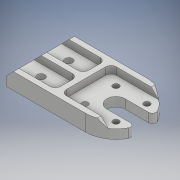
# Autodesk Inventor part: holder-LMF8LUU-z-axis-v2
Saved by Autodesk Inventor 2018 (Build 220112000, 112)
## iProperties
Created: 2017-12-27
Part Number: holder-LMF8LUU-z-axis-v2
Material: Generic
Document SubType Name: Modeling
Designer: Jurjen
Density: 1 g/cm^3
Appearance: Default
Author: Jurjen
Autodesk Inventor part; units mm, degrees
ref_plane "YZ Plane" through (0, 0, 0) normal (1, 0, 0) x (0, 1, 0)
ref_plane "XZ Plane" through (0, 0, 0) normal (0, 1, 0) x (-1, 0, 0)
ref_plane "XY Plane" through (0, 0, 0) normal (0, 0, 1) x (1, 0, 0)
sketch "Sketch1" plane through (0, 0, 0) normal (0, 0, 1) x (1, 0, 0)
  arc A0 (13.75, 5) -> (13.75, -5) centre (13.75, 0) ccw
  line L0 (29.75, 16.75) -> (-29.75, 16.75)
  line L1 (-29.75, 16.75) -> (-29.75, -16.75)
  line L2 (-29.75, -16.75) -> (29.75, -16.75)
  line L3 (29.75, -16.75) -> (29.75, 16.75)
  line L4 (13.75, 5) -> (29.75, 5)
  line L5 (13.75, -5) -> (29.75, -5)
  arc A1 (13.75, -5) -> (13.75, 5) centre (13.75, 0) ccw construction
  point P0 (0, 0)
  point P1 (0, -16.75)
  point P2 (29.75, 0)
  point P3 (-29.75, 0)
  dimension "d0" = 10
  dimension "d1" = 33.5
  dimension "d2" = 16
  dimension "d3" = 43.5
  constraints: 12 end point, 4 point on circle, 3 midpoint, 3 perpendicular, 2 centre point, 2 horizontal alignment, 2 parallel, 2 point on line, 2 tangent, 1 horizontal, 1 vertical alignment
  measures "d0" diameter of A0
  measures "d1" distance between parallel lines of L2 L0
  measures "d2" distance from line of L3 A0.centre
  measures "d3" distance from line of L1 A0.centre
extrude "Extrusion1" add sketch "Sketch1" along normal mid plane 5 contours A0 L5 L3 L2 L1 L0 L4
sketch "Sketch2" plane through (0, 0, 2.5) normal (0, 0, 1) x (1, 0, 0)
  arc A0 (13.75, 5) -> (13.75, -5) centre (13.75, 0) ccw projected
  circle A1 centre (5.2647, 8.4853) radius 1.65
  line L0 (13.75, 0) -> (5.2647, 8.4853) construction
  line L1 (13.75, 0) -> (0, 0) construction
  line L2 (13.75, 0) -> (13.75, -13.75) construction
  circle A2 centre (5.2647, -8.4853) radius 1.65
  line L3 (13.75, 0) -> (27.5, 0) construction
  circle A3 centre (22.2353, -8.4853) radius 1.65
  line L4 (13.75, 0) -> (13.75, 13.75) construction
  circle A4 centre (22.2353, 8.4853) radius 1.65
  dimension "d6" = 45
  dimension "d7" = 12
  dimension "d8" = 3.3
  dimension "d11" = 360
  constraints: 10 end point, 4 centre point, 2 coincident, 1 horizontal, 19 other
  measures "d6" angle of L1 L0
  measures "d7" distance of L0.start L0.end
  measures "d8" diameter of A1
extrude "Extrusion2" cut sketch "Sketch2" against normal through all
sketch "Sketch3" plane through (0, 0, 2.5) normal (0, 0, 1) x (1, 0, 0)
  circle A0 centre (-19.75, 7.625) radius 2.1
  line L0 (0, 0) -> (-29.75, 0) construction
  line L1 (-29.75, 16.75) -> (-29.75, -16.75) projected
  circle A1 centre (-19.75, -7.625) radius 2.1
  dimension "d15" = 4.2
  dimension "d16" = 10
  dimension "d37" = 9.125
  constraints: 2 centre point, 2 end point, 1 midpoint, 1 symmetric about line, 1 other
  measures "d15" diameter of A0
  measures "d16" distance from line of A0.centre L1
  measures "d37" vertical distance of A0.centre L1.start
extrude "Extrusion3" cut sketch "Sketch3" against normal through all
sketch "Sketch4" plane through (0, 0, 2.5) normal (0, 0, 1) x (1, 0, 0)
  line L0 (-29.75, 16.75) -> (29.75, 16.75) projected
  line L1 (-29.75, 16.75) -> (29.75, 16.75)
  line L2 (29.75, 16.75) -> (29.75, 13.75)
  line L3 (-29.75, 13.75) -> (-29.75, 16.75)
  line L4 (-2.75, 13.75) -> (-2.75, 0)
  line L5 (-5.75, 1.5) -> (-5.75, 13.75)
  line L6 (-29.75, 1.5) -> (-5.75, 1.5)
  line L7 (-29.75, 0) -> (-29.75, 1.5)
  line L8 (29.75, 13.75) -> (-2.75, 13.75)
  line L9 (-5.75, 13.75) -> (-29.75, 13.75)
  line L10 (0, 0) -> (-29.75, 0) construction
  line L11 (-29.75, -16.75) -> (-29.75, 16.75) projected
  line L12 (-29.75, -16.75) -> (29.75, -16.75)
  line L13 (-29.75, -16.75) -> (29.75, -16.75)
  line L14 (29.75, -16.75) -> (29.75, -13.75)
  line L15 (-29.75, -13.75) -> (-29.75, -16.75)
  line L16 (-2.75, -13.75) -> (-2.75, 0)
  line L17 (-5.75, -1.5) -> (-5.75, -13.75)
  line L18 (-29.75, -1.5) -> (-5.75, -1.5)
  line L19 (-29.75, 0) -> (-29.75, -1.5)
  line L20 (29.75, -13.75) -> (-2.75, -13.75)
  line L21 (-5.75, -13.75) -> (-29.75, -13.75)
  point P0 (29.75, 5)
  dimension "d20" = 3
  dimension "d21" = 3
  dimension "d23" = 24
  dimension "d24" = 1.5
  constraints: 40 end point, 8 symmetric about line, 5 parallel, 3 horizontal alignment, 3 perpendicular, 2 horizontal, 2 point on line, 2 vertical alignment
  measures "d20" distance between parallel lines of L0 L8
  measures "d21" distance between parallel lines of L4 L5
  measures "d23" distance of L5.end L3.start
  measures "d24" distance of L7.start L6.start
extrude "Extrusion4" add sketch "Sketch4" along normal blind 4 contours L0 L2 L8 L4 L16 L20 L14 L12 L11 L21 L17 L18 L7 L6 L5 L9 L3
sketch "Sketch5" plane through (0, 0, -2.5) normal (0, 0, -1) x (-1, 0, 0)
  arc A0 (-13.75, -5) -> (-13.75, 5) centre (-13.75, 0) ccw projected
  line L0 (29.75, 16.75) -> (-29.75, 16.75) projected
  circle A1 centre (19.75, 7.625) radius 2.1 projected
  circle A2 centre (19.75, -7.625) radius 2.1 projected
  circle A3 centre (-22.2353, -8.4853) radius 1.65 projected
  circle A4 centre (-5.2647, 8.4853) radius 1.65 projected
  circle A5 centre (-5.2647, -8.4853) radius 1.65 projected
  circle A6 centre (-22.2353, 8.4853) radius 1.65 projected
  line L1 (29.75, 16.75) -> (-29.75, 16.75) projected
  line L2 (-29.75, 16.75) -> (-29.75, 5) projected
  line L3 (-29.75, 5) -> (-13.75, 5) projected
  arc A7 (-13.75, -5) -> (-13.75, 5) centre (-13.75, 0) ccw projected
  line L4 (-13.75, -5) -> (-29.75, -5) projected
  line L5 (-29.75, -5) -> (-29.75, -16.75) projected
  line L6 (-29.75, -16.75) -> (29.75, -16.75) projected
  line L7 (29.75, -16.75) -> (29.75, 16.75) projected
  line L8 (-13.75, -16.75) -> (-29.75, -16.75)
  line L9 (-29.75, -13.75) -> (-29.75, -5) projected
  line L10 (-29.75, -5) -> (-29.75, -16.75)
  line L11 (-29.75, 5) -> (-29.75, 16.75)
  line L12 (-13.75, 16.75) -> (-29.75, 16.75)
  arc A8 (-13.75, 16.75) -> (-29.7363, 5) centre (-13.75, 0) ccw
  arc A9 (-29.7363, -5) -> (-13.75, -16.75) centre (-13.75, 0) ccw
  point P0 (0, 0)
  constraints: 8 end point, 4 point on circle, 4 point on line, 3 collinear, 2 centre point, 2 tangent, 1 coincident, 1 perpendicular
extrude "Extrusion5" cut sketch "Sketch5" against normal through all contours A9 L6 L5 L4 | L3 L2 L0 A8
fillet "Fillet1" radius 2 2 edges at (29.7363, -5, 0) (29.7363, 5, 0)
chamfer "Chamfer1" distance 4 angle 45 3 edges at (-29.75, 15.25, 6.5) (-29.75, 0, 6.5) (-29.75, -15.25, 6.5)
sketch "Sketch6" plane through (-29.75, -16.75, -2.5) normal (0, -1, 0) x (1, 0, 0)
  line L0 (58.2436, 5) -> (58.2436, 0) projected
  line L1 (53.0656, 5) -> (58.2436, 5) projected
  line L2 (53.0656, 9) -> (53.0656, 5) projected
  line L3 (43.5, 9) -> (53.0656, 9) projected
  line L4 (43.5, 9) -> (43.5, 0) projected
  line L5 (58.2436, 0) -> (43.5, 0) projected
  line L6 (53.0656, 5) -> (49.0656, 9)
  line L7 (27, 9) -> (53.0656, 9) projected
  line L8 (53.0656, 9) -> (27, 9) projected
  line L9 (49.0656, 9) -> (53.0656, 9)
  line L10 (53.0656, 9) -> (53.0656, 5)
  point P0 (29.75, 2.5)
  dimension "d33" = 45
  constraints: 6 end point, 1 collinear, 1 perpendicular, 1 point on line
  measures "d33" angle of L3 L6
extrude "Extrusion6" cut sketch "Sketch6" against normal through all contours L6 L3 L2
fillet "Fillet2" radius 3 6 edges at (-2.75, -13.75, 4.5) (-5.75, -13.75, 4.5) (-2.75, 13.75, 4.5) (-5.75, -1.5, 4.5) (-5.75, 13.75, 4.5) (-5.75, 1.5, 4.5)
equation "\"d21\" = d20"
equation "\"d24\" = 0.5 * d20"
body "Solid1"
